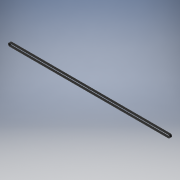
# Autodesk Inventor part: GBN9942GT-60_.info-1-14-14
Saved by Autodesk Inventor 2019 (Build 230136000, 136)
## iProperties
Created: 2022-10-05
Part Number: GBN9942GT-60_.info-1-14-14
Material: Generic
Catalog Web Link: www.cadenas.de
Description: GBN__2GT-High Torque Timing Belts 2GT
Vendor: MISUMI
Document SubType Name: Modeling
Designer: psAdmin
Manufacturer: MISUMI
Mass: 3.78054 g
Surface Area: 132.177 cm^2
Volume: 3.78054 cm^3
Density: 1 g/cm^3
Appearance: PSOLRGB-175-175-175
Category: PARTsolutions
Company: MISUMI
Title: GBN9942GT-60
Author: Cadenas PARTsolutions
Comments: High Torque Timing Belts 2GT
PSOL_IDENT_0: {$CADENAS_DATA/23d-libs/misumi/metric/48_timing_belts/gbn_gt2.prj},205 {VTYP=3D},{NB=GBN9942GT-60_.i
PSOL_IDENT_1: nfo-1-14-14},{LINA=GBN9942GT-60},{NN=GBN__2GT},{DATE=08.06.2021 08:28:53},{GEOMDATE=01.05.2017 02:05
PSOL_IDENT_2: :38},{VERSION=},{LINEID=50},{WBVAR=NT,RSSP,NT1,NT2},{WBNUMERIC=NT,NT1,NT2}  {NB=GBN9942GT-60_.info-1
PSOL_IDENT_3: -14-14},{LINA=GBN9942GT-60},{KT=DUMMY},{PN=GBN9942GT-60},{TYPE=GBN},{BNO=9942GT},{BNW=6},{NT=497},{N
PSOL_IDENT_4: TALG=33,36,37,38,39,40,41,42,43,44,45,46,47,48,49,50,51,53,54,55,56,57,58,59,60,61,62,63,64,65,66,67
PSOL_IDENT_5: ,68,69,70,71,72,73,74,75,76,77,78,79,80,81,82,83,84,85,86,87,88,89,90,91,92,93,94,95,96,97,98,100,10
PSOL_IDENT_6: 1,102,104,105,106,107,108,110,112,113,114,115,116,118,120,121,122,124,125,126,127,128,129,130,132,13
PSOL_IDENT_7: 3,134,135,139,140,141,142,143,144,145,146,147,150,151,152,154,155,157,159,160,161,162,163,164,166,16
PSOL_IDENT_8: 8,169,170,172,173,174,175,176,177,179,180,183,185,186,188,190,191,193,197,200,203,206,210,213,215,21
PSOL_IDENT_9: 8,220,222,223,224,226,230,235,239,242,243,244,246,247,250,251,252,253,258,262,265,272,275,279,285,28
PSOL_IDENT_10: 6,289,293,299,300,303,308,315,317,323,330,335,338,345,348,351,363,371,376,380,386,391,400,405,426,43
PSOL_IDENT_11: 0,433,446,450,465,475,488,497},{BC=994},{PITCH=2},{R1=0.15},{R2=1},{R3=0.555},{BB=0.4},{H=1.38},{HH=
PSOL_IDENT_12: 0.75},{II=0.63},{PLD=0.254},{RSSP=1},{RSSPALG= '1','900 or Less','2','Over 900, 1200 or Less','3','O
PSOL_IDENT_13: ver 1200, 1800 or Less','4','Over 1800, 3600 or Less','5','Over 3600, 4800 or Less' },{NT1=14},{NT1A
PSOL_IDENT_14: LG=14,15,16,18,20,21,22,24,25,26,28,30,32,34,36,38,40,44,48,50,60},{NT2=14},{NT2ALG=14,15,16,18,20,2
PSOL_IDENT_15: 1,22,24,25,26,28,30,32,34,36,38,40,44,48,50,60},{DRIVEP=8.91268},{DRP=8.4},{DRIVENP=8.91268},{DRNP=8
PSOL_IDENT_16: .4},{BBCAL=1932.00000},{C=483.00},{NOTE=-},{FS=13.00},{FL=13.00}
NB: GBN9942GT-60_.info-1-14-14
NN: GBN__2GT
NT: 497
NBSYN: $PN._.info-$RSSP.-$NT1.-$NT2.
LINA: GBN9942GT-60
CATALOG: Misumi
PN: GBN9942GT-60
BNO: 9942GT
BNW: 6
PITCH: 2
R1: 0.15
R2: 1
R3: 0.555
BB: 0.4
H: 1.38
HH: 0.75
II: 0.63
PLD: 0.254
RSSP: 900 or Less
NT1: 14
NT2: 14
NOTE: -
SUPPLIER: MISUMI
ARTICLENO: GBN9942GT-60_.info-1-14-14
BOMINFO: GBN9942GT-60
CREATOR: CADENAS GmbH
Autodesk Inventor part; units mm, degrees
ref_plane "YZ Plane" through (0, 0, 0) normal (1, 0, 0) x (0, 1, 0)
ref_plane "XZ Plane" through (0, 0, 0) normal (0, 1, 0) x (-1, 0, 0)
ref_plane "XY Plane" through (0, 0, 0) normal (0, 0, 1) x (1, 0, 0)
sketch "_____1" plane through (0, 0, 0) normal (0, 0, 1) x (1, 0, 0)
  arc A0 (0, 4.83) -> (0, -4.83) centre (0, 0) ccw
  line L0 (0, -4.83) -> (483, -4.83)
  arc A1 (483, -4.83) -> (483, 4.83) centre (483, 0) ccw
  line L1 (483, 4.83) -> (0, 4.83)
  arc A2 (0, 4.2) -> (0, -4.2) centre (0, 0) ccw
  line L2 (0, -4.2) -> (483, -4.2)
  arc A3 (483, -4.2) -> (483, 4.2) centre (483, 0) ccw
  line L3 (483, 4.2) -> (0, 4.2)
  constraints: 8 end point, 8 point on circle, 4 centre point
extrude "Extrusion1" add sketch "_____1" along normal mid plane 6
sketch "_____2" plane through (0, 0, 0) normal (0, 0, 1) x (1, 0, 0)
  line L0 (236.5, 4.83) -> (236.5, 4.2)
  line L1 (236.5, 4.2) -> (236.7598, 4.2)
  arc A0 (236.9085, 4.0696) -> (236.7598, 4.2) centre (236.7598, 4.05) ccw
  arc A1 (236.9085, 4.0696) -> (237.0011, 3.7618) centre (237.9, 4.2) ccw
  arc A2 (237.0011, 3.7618) -> (237.9989, 3.7618) centre (237.5, 4.005) ccw
  arc A3 (237.9989, 3.7618) -> (238.0915, 4.0696) centre (237.1, 4.2) ccw
  arc A4 (238.2402, 4.2) -> (238.0915, 4.0696) centre (238.2402, 4.05) ccw
  line L2 (238.2402, 4.2) -> (238.7598, 4.2)
  arc A5 (238.9085, 4.0696) -> (238.7598, 4.2) centre (238.7598, 4.05) ccw
  arc A6 (238.9085, 4.0696) -> (239.0011, 3.7618) centre (239.9, 4.2) ccw
  arc A7 (239.0011, 3.7618) -> (239.9989, 3.7618) centre (239.5, 4.005) ccw
  arc A8 (239.9989, 3.7618) -> (240.0915, 4.0696) centre (239.1, 4.2) ccw
  arc A9 (240.2402, 4.2) -> (240.0915, 4.0696) centre (240.2402, 4.05) ccw
  line L3 (240.2402, 4.2) -> (240.7598, 4.2)
  arc A10 (240.9085, 4.0696) -> (240.7598, 4.2) centre (240.7598, 4.05) ccw
  arc A11 (240.9085, 4.0696) -> (241.0011, 3.7618) centre (241.9, 4.2) ccw
  arc A12 (241.0011, 3.7618) -> (241.9989, 3.7618) centre (241.5, 4.005) ccw
  arc A13 (241.9989, 3.7618) -> (242.0915, 4.0696) centre (241.1, 4.2) ccw
  arc A14 (242.2402, 4.2) -> (242.0915, 4.0696) centre (242.2402, 4.05) ccw
  line L4 (242.2402, 4.2) -> (242.7598, 4.2)
  arc A15 (242.9085, 4.0696) -> (242.7598, 4.2) centre (242.7598, 4.05) ccw
  arc A16 (242.9085, 4.0696) -> (243.0011, 3.7618) centre (243.9, 4.2) ccw
  arc A17 (243.0011, 3.7618) -> (243.9989, 3.7618) centre (243.5, 4.005) ccw
  arc A18 (243.9989, 3.7618) -> (244.0915, 4.0696) centre (243.1, 4.2) ccw
  arc A19 (244.2402, 4.2) -> (244.0915, 4.0696) centre (244.2402, 4.05) ccw
  line L5 (244.2402, 4.2) -> (244.7598, 4.2)
  arc A20 (244.9085, 4.0696) -> (244.7598, 4.2) centre (244.7598, 4.05) ccw
  arc A21 (244.9085, 4.0696) -> (245.0011, 3.7618) centre (245.9, 4.2) ccw
  arc A22 (245.0011, 3.7618) -> (245.9989, 3.7618) centre (245.5, 4.005) ccw
  arc A23 (245.9989, 3.7618) -> (246.0915, 4.0696) centre (245.1, 4.2) ccw
  arc A24 (246.2402, 4.2) -> (246.0915, 4.0696) centre (246.2402, 4.05) ccw
  line L6 (246.2402, 4.2) -> (246.5, 4.2)
  line L7 (246.5, 4.2) -> (246.5, 4.83)
  line L8 (246.5, 4.83) -> (236.5, 4.83)
  constraints: 50 point on circle, 25 centre point, 18 end point
extrude "Extrusion2" add sketch "_____2" along normal mid plane 6
body "Solid1"
